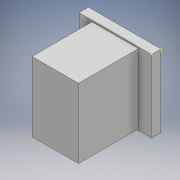
# Autodesk Inventor part: CRANEBASE
Saved by Autodesk Inventor 2017 (Build 210142000, 142)
## iProperties
Part Number: CRANEBASE
Material: 一般
Document SubType Name: Modeling
Designer: rsdlab
Density: 1 g/cm^3
Appearance: 既定
Author: rsdlab
Autodesk Inventor part; units mm, degrees
ref_plane "YZ Plane" through (0, 0, 0) normal (1, 0, 0) x (0, 1, 0)
ref_plane "XZ Plane" through (0, 0, 0) normal (0, 1, 0) x (-1, 0, 0)
ref_plane "XY Plane" through (0, 0, 0) normal (0, 0, 1) x (1, 0, 0)
sketch "スケッチ1" plane through (0, 0, 0) normal (0, 1, 0) x (-1, 0, 0)
  line L0 (0, 0) -> (0.5, 0)
  line L1 (0.5, 0) -> (0.5, -0.5)
  line L2 (0.5, -0.5) -> (0, -0.5)
  line L3 (0, -0.5) -> (0, 0)
  dimension "d0" = 0.5
  dimension "d1" = 0.5
  constraints: 8 end point, 2 parallel, 1 horizontal, 1 perpendicular
  measures "d0" distance of L1.end L2.end
  measures "d1" distance of L0.end L1.end
extrude "押し出し1" add sketch "スケッチ1" against normal blind 0.065
sketch "スケッチ2" plane through (0, -0.065, 0) normal (0, -1, 0) x (1, 0, 0)
  point P0 (0, 0)
sketch "スケッチ3" plane through (0, -0.065, 0) normal (0, -1, 0) x (1, 0, 0)
  line L0 (0, 0) -> (-0.5, 0) projected
  line L1 (-0.5, -0.5) -> (0, -0.5) projected
  line L2 (-0.09, -0.01) -> (-0.41, -0.01)
  line L3 (-0.41, -0.01) -> (-0.41, -0.49)
  line L4 (-0.41, -0.49) -> (-0.09, -0.49)
  line L5 (-0.09, -0.49) -> (-0.09, -0.01)
  point P0 (-0.09, 0)
  point P1 (-0.41, -0.5)
  dimension "d7" = 0.32
  dimension "d8" = 0.48
  constraints: 8 end point, 2 parallel, 2 point on line, 1 horizontal, 1 perpendicular
  measures "d7" distance of L4.end L3.end
  measures "d8" distance of L3.end L2.end
extrude "押し出し2" add sketch "スケッチ3" along normal blind 0.414
sketch "スケッチ4" plane through (0, 0, 0) normal (1, 0, 0) x (0, 0, -1)
  point P0 (0, 0)
sketch "スケッチ5" plane through (0, -0.065, 0) normal (0, -1, 0) x (1, 0, 0)
  point P0 (0, 0)
sketch "スケッチ6" plane through (-0.41, -0.065, -0.01) normal (0, 0, 1) x (1, 0, 0)
  point P0 (0.41, 0.065)
